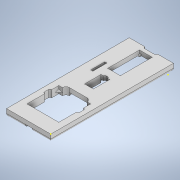
# Autodesk Inventor part: inside
Saved by Autodesk Inventor 2022 (Build 260153000, 153)
## iProperties
Created: 2022-12-24
Part Number: inside
Material: Generic
Document SubType Name: Modeling
Designer: matys
Density: 1 g/cm^3
Appearance: Default
Author: matys
Autodesk Inventor part; units mm, degrees
ref_plane "YZ Plane" through (0, 0, 0) normal (1, 0, 0) x (0, 1, 0)
ref_plane "XZ Plane" through (0, 0, 0) normal (0, 1, 0) x (-1, 0, 0)
sketch "Sketch1" plane through (0, 0, 0) normal (0, 1, 0) x (-1, 0, 0)
  line L0 (0, 0) -> (0, -173.4)
  line L1 (0, -173.4) -> (62.5, -173.4)
  line L2 (62.5, -173.4) -> (62.5, 0)
  line L3 (62.5, 0) -> (0, 0)
  dimension "d0" = 173.4
  dimension "d1" = 62.5
  constraints: 8 end point, 3 perpendicular, 1 vertical
  measures "d0" distance of L0.start L0.end
  measures "d1" distance of L0.end L1.end
extrude "Extrusion1" add sketch "Sketch1" along normal blind 10
sketch "Sketch2" plane through (0, 10, 0) normal (0, 1, 0) x (1, 0, 0)
  line L0 (0, 0) -> (0, 102.12)
  line L1 (0, 0) -> (0, 173.4) projected
  line L2 (0, 102.12) -> (-62.5, 102.12)
  line L3 (-62.5, 173.4) -> (-62.5, 0) projected
  line L4 (-31.25, 102.12) -> (-31.25, 0)
  line L5 (-62.5, 0) -> (0, 0) projected
  line L6 (-31.25, 102.12) -> (-37.45, 102.12)
  line L7 (-37.45, 102.12) -> (-31.25, 102.12)
  line L8 (-31.25, 102.12) -> (-25.05, 102.12)
  line L9 (-25.05, 102.12) -> (-31.25, 102.12)
  line L10 (-31.25, 102.12) -> (-31.25, 85.22)
  line L11 (-31.25, 85.22) -> (-25.05, 85.22)
  line L12 (-25.05, 85.22) -> (-25.05, 102.12)
  line L13 (-31.25, 85.22) -> (-37.45, 85.22)
  line L14 (-37.45, 85.22) -> (-37.45, 102.12)
  line L15 (-31.25, 102.12) -> (-31.25, 108.42)
  line L16 (-31.25, 108.42) -> (-25.05, 108.42)
  line L17 (-25.05, 108.42) -> (-25.05, 102.12)
  line L18 (-37.45, 102.12) -> (-37.45, 108.42)
  line L19 (-37.45, 108.42) -> (-31.25, 108.42)
  line L20 (-31.25, 108.42) -> (-31.25, 173.4)
  line L21 (0, 173.4) -> (-62.5, 173.4) projected
  line L22 (-31.25, 140.91) -> (-31.25, 120.66)
  line L23 (-31.25, 120.66) -> (-22.25, 120.66)
  line L24 (-22.25, 120.66) -> (-22.25, 165.66)
  line L25 (-22.25, 165.66) -> (-40.25, 165.66)
  line L26 (-40.25, 165.66) -> (-40.25, 120.66)
  line L27 (-40.25, 120.66) -> (-31.25, 120.66)
  line L28 (-40.25, 120.66) -> (-40.25, 126.66)
  line L29 (-40.25, 126.66) -> (-44.25, 126.66)
  line L30 (-44.25, 126.66) -> (-47.25, 126.66)
  line L31 (-47.25, 126.66) -> (-47.25, 106.66)
  line L32 (-47.25, 106.66) -> (-50.25, 106.66)
  line L33 (-50.25, 106.66) -> (-50.25, 126.66)
  line L34 (-50.25, 126.66) -> (-47.25, 126.66)
  line L35 (-31.25, 0) -> (-31.25, 85.22)
  line L36 (-31.25, 42.61) -> (-31.25, 20.11)
  line L37 (-31.25, 20.11) -> (-31.25, 42.61)
  line L38 (-31.25, 42.61) -> (-31.25, 65.11)
  line L39 (-31.25, 65.11) -> (-53.75, 65.11)
  line L40 (-53.75, 65.11) -> (-53.75, 20.11)
  line L41 (-53.75, 20.11) -> (-8.75, 20.11)
  line L42 (-8.75, 20.11) -> (-8.75, 65.11)
  line L43 (-8.75, 65.11) -> (-31.25, 65.11)
  line L44 (-22.25, 120.66) -> (-40.25, 120.66)
  line L45 (-40.25, 120.66) -> (-40.25, 165.66)
  line L46 (-40.25, 165.66) -> (-22.25, 165.66)
  line L47 (-22.25, 165.66) -> (-22.25, 120.66)
  line L48 (-53.75, 65.11) -> (-48.75, 65.11)
  line L49 (-48.75, 65.11) -> (-8.75, 65.11)
  line L50 (-8.75, 65.11) -> (-13.75, 65.11)
  line L51 (-13.75, 65.11) -> (-13.75, 70.11)
  line L52 (-13.75, 70.11) -> (-48.75, 70.11)
  line L53 (-48.75, 70.11) -> (-48.75, 65.11)
  line L54 (-48.75, 65.11) -> (-13.75, 65.11) construction
  line L55 (-18.75, 70.11) -> (-43.75, 70.11)
  arc A0 (-43.75, 70.11) -> (-48.75, 65.11) centre (-43.75, 65.11) ccw
  arc A1 (-13.75, 65.11) -> (-18.75, 70.11) centre (-18.75, 65.11) ccw
  line L56 (-8.75, 65.11) -> (-8.75, 55.11)
  line L57 (-8.75, 55.11) -> (-8.75, 45.11)
  line L58 (-8.75, 45.11) -> (-53.75, 45.11)
  line L59 (-53.75, 45.11) -> (-53.75, 55.11)
  line L60 (-53.75, 45.11) -> (-53.75, 55.11) construction
  line L61 (-51.25, 47.61) -> (-51.25, 52.61)
  line L62 (-56.25, 52.61) -> (-56.25, 47.61)
  arc A2 (-56.25, 47.61) -> (-51.25, 47.61) centre (-53.75, 47.61) ccw
  arc A3 (-51.25, 52.61) -> (-56.25, 52.61) centre (-53.75, 52.61) ccw
  line L63 (-8.75, 45.11) -> (-8.75, 55.11) construction
  line L64 (-6.25, 47.61) -> (-6.25, 52.61)
  line L65 (-11.25, 52.61) -> (-11.25, 47.61)
  arc A4 (-11.25, 47.61) -> (-6.25, 47.61) centre (-8.75, 47.61) ccw
  arc A5 (-6.25, 52.61) -> (-11.25, 52.61) centre (-8.75, 52.61) ccw
  line L66 (-40.25, 165.66) -> (-40.25, 173.4)
  line L67 (-22.25, 165.66) -> (-22.25, 173.4)
  line L68 (-40.25, 173.4) -> (-22.25, 173.4) construction
  line L69 (-37.75, 170.9) -> (-24.75, 170.9)
  line L70 (-24.75, 175.9) -> (-37.75, 175.9)
  arc A6 (-37.75, 175.9) -> (-37.75, 170.9) centre (-37.75, 173.4) ccw
  arc A7 (-24.75, 170.9) -> (-24.75, 175.9) centre (-24.75, 173.4) ccw
  line L71 (-31.25, 102.12) -> (-34.35, 102.12)
  line L72 (-28.15, 102.12) -> (-31.25, 102.12)
  line L73 (-34.35, 102.12) -> (-28.15, 102.12) construction
  line L74 (-32.35, 100.12) -> (-30.15, 100.12)
  line L75 (-30.15, 104.12) -> (-32.35, 104.12)
  arc A8 (-32.35, 104.12) -> (-32.35, 100.12) centre (-32.35, 102.12) ccw
  arc A9 (-30.15, 100.12) -> (-30.15, 104.12) centre (-30.15, 102.12) ccw
  arc A10 (-32.35, 110.42) -> (-32.35, 106.42) centre (-32.35, 108.42) ccw
  arc A11 (-30.15, 106.42) -> (-30.15, 110.42) centre (-30.15, 108.42) ccw
  line L76 (-32.35, 110.42) -> (-30.15, 110.42)
  point P0 (-31.25, 165.66)
  point P1 (-31.25, 165.66)
  point P2 (-53.75, 50.11)
  point P3 (-8.75, 50.11)
  point P4 (-34.35, 108.42)
  point P5 (-28.15, 108.42)
  dimension "d4" = 102.12
  dimension "d5" = 6.2
  dimension "d6" = 6.2
  dimension "d7" = 16.9
  dimension "d8" = 6.3
  dimension "d11" = 20.25
  dimension "d12" = 9
  dimension "d13" = 45
  dimension "d14" = 18
  dimension "d15" = 6
  dimension "d16" = 4
  dimension "d17" = 3
  dimension "d18" = 20
  dimension "d19" = 3
  dimension "d20" = 22.5
  dimension "d21" = 22.5
  dimension "d22" = 22.5
  dimension "d23" = 45
  dimension "d24" = 5
  dimension "d25" = 5
  dimension "d26" = 5
  dimension "d27" = 10
  dimension "d28" = 10
  dimension "d29" = 5
  dimension "d30" = 5
  dimension "d36" = 5
  dimension "d37" = 4
  dimension "d39" = 4
  constraints: 156 end point, 35 point on circle, 33 point on line, 30 perpendicular, 18 tangent, 12 centre point, 12 midpoint, 7 collinear, 7 parallel, 4 horizontal, 1 vertical
  measures "d4" distance of L0.start L0.end
  measures "d5" distance of L4.start L6.end
  measures "d6" distance of L4.start L8.end
  measures "d7" distance of L4.start L10.end
  measures "d8" distance of L4.start L15.end
  measures "d11" distance of L22.start L22.end
  measures "d12" distance of L22.end L23.end
  measures "d13" distance of L23.end L24.end
  measures "d14" distance of L24.end L25.end
  measures "d15" distance of L26.end L28.end
  measures "d16" distance of L28.end L29.end
  measures "d17" distance of L29.end L30.end
  measures "d18" distance of L30.end L31.end
  measures "d19" distance of L31.end L32.end
  measures "d20" distance of L36.start L36.end
  measures "d21" distance of L36.start L38.end
  measures "d22" distance of L38.end L39.end
  measures "d23" distance of L40.end L41.end
  measures "d24" distance of L48.end L39.end
  measures "d25" distance of L50.end L42.end
  measures "d26" distance of L50.end L51.end
  measures "d27" distance of L42.end L56.end
  measures "d28" distance of L56.end L57.end
  measures "d29" diameter of A3
  measures "d30" diameter of A5
  measures "d36" diameter of A7
  measures "d37" diameter of A9
  measures "d39" diameter of A11
extrude "Extrusion2" cut sketch "Sketch2" against normal through all contours L12 L11 L4 L74 A9 L2 | L2 A9 L75 L15 L16 L17 | L41 L40 L58 L4 | L4 L58 L42 L41 | A7 L69 L20 L21 | A9 L74 L4 L2 | L2 L15 L75 A9 | L31 L32 L33 L34 | L20 L69 A6 L21 | L24 L23 L20 L25 | L4 L74 A8 L2 | L2 A8 L75 L15 | L13 L14 L2 A8 L74 L4 | L16 L20 L76 A11 | L58 A2 L61 A3 L40 L39 L4 | L4 L43 L42 A5 L65 A4 L58 | A2 L62 A3 L40 | L40 A3 L61 A2 | A4 L65 A5 L42 | L42 A5 L64 A4 | L18 L19 L15 L75 A8 L2 | L20 L27 L26 L25 | L52 A1 L43 L4 | L4 L39 A0 L52 | L19 A10 L76 L20
sketch "Sketch3" plane through (0, 10, 0) normal (0, 1, 0) x (1, 0, 0)
  point P0 (0, 0)
sketch "Sketch4" plane through (0, 0, 0) normal (0, -1, 0) x (1, 0, 0)
  line L0 (-8.75, -20.11) -> (-53.75, -20.11) projected
  line L1 (-53.75, -20.11) -> (-8.75, -20.11)
  line L2 (-8.75, -20.11) -> (-31.25, -20.11)
  line L3 (-62.5, 0) -> (0, 0) projected
  line L4 (-31.25, 0) -> (-31.25, -20.11)
  line L5 (-31.25, -20.11) -> (-26.25, -20.11)
  line L6 (-26.25, -20.11) -> (-36.25, -20.11)
  line L7 (-36.25, -20.11) -> (-36.25, 0)
  line L8 (-36.25, 0) -> (-26.25, 0)
  line L9 (-26.25, 0) -> (-26.25, -20.11)
  line L10 (-40.25, -165.66) -> (-40.25, -120.66) projected
  line L11 (-40.25, -120.66) -> (-47.25, -120.66)
  line L12 (-47.25, -126.66) -> (-47.25, -106.66) projected
  line L13 (-48.8082, -126.9328) -> (-40.25, -126.9328)
  line L14 (-40.25, -126.9328) -> (-48.8082, -126.9328)
  line L15 (-40.25, -165.66) -> (-22.25, -165.66) projected
  line L16 (-40.25, -165.66) -> (-48.8082, -165.66)
  line L17 (-48.8082, -165.66) -> (-48.8082, -126.9328)
  line L18 (-22.25, -120.66) -> (-22.25, -165.66) projected
  line L19 (-22.25, -165.66) -> (-15.25, -165.66)
  line L20 (-15.25, -165.66) -> (-15.25, -120.66)
  line L21 (-15.25, -120.66) -> (-22.25, -120.66)
  line L22 (-40.25, -120.66) -> (-22.25, -120.66) projected
  line L23 (-22.25, -120.66) -> (-40.25, -120.66)
  line L24 (-40.25, -120.66) -> (-40.25, -126.9328)
  line L25 (-40.25, -165.66) -> (-40.25, -126.9328)
  line L26 (-22.25, -120.66) -> (-22.25, -165.66)
  line L27 (-40.25, -165.66) -> (-40.25, -173.4)
  line L28 (0, -173.4) -> (-62.5, -173.4) projected
  line L29 (-48.8082, -165.66) -> (-40.25, -173.4)
  line L30 (-22.25, -165.66) -> (-22.25, -173.4)
  line L31 (-22.25, -173.4) -> (-15.25, -165.66)
  line L32 (-40.25, -173.4) -> (-22.25, -173.4)
  line L33 (-37.45, -108.42) -> (-37.45, -85.22) projected
  line L34 (-25.05, -85.22) -> (-25.05, -108.42) projected
  line L35 (-37.45, -108.42) -> (-25.05, -108.42)
  line L36 (-25.05, -108.42) -> (-22.25, -120.66)
  line L37 (-37.45, -108.42) -> (-40.25, -120.66)
  line L38 (-43.75, -70.11) -> (-18.75, -70.11) projected
  line L39 (-50.25, -126.66) -> (-50.25, -106.66) projected
  line L40 (-43.75, -70.11) -> (-50.25, -106.66)
  line L41 (-47.25, -106.66) -> (-50.25, -106.66) projected
  line L42 (-47.25, -106.66) -> (-40.25, -70.11)
  line L43 (-18.75, -70.11) -> (-15.25, -120.66)
  line L44 (-25.05, -108.42) -> (-37.45, -108.42) projected
  line L45 (-25.05, -85.22) -> (-37.45, -85.22) projected
  line L46 (-25.05, -108.42) -> (-25.05, -85.22)
  line L47 (-25.05, -85.22) -> (-43.1438, -85.22)
  line L48 (-37.45, -108.42) -> (-47.25, -120.66)
  line L49 (-48.8082, -126.9328) -> (-48.8082, -120.66)
  line L50 (-48.8082, -120.66) -> (-47.25, -120.66)
  line L51 (-37.45, -108.42) -> (-47.25, -108.42)
  line L52 (-37.45, -108.42) -> (-38.0612, -111.0919)
  line L53 (-38.0612, -111.0919) -> (-47.25, -111.0919)
  point P0 (-39.5893, -111.0919)
  dimension "d31" = 5
  dimension "d32" = 10
  dimension "d33" = 7
  constraints: 78 end point, 14 perpendicular, 13 point on line, 4 horizontal, 3 collinear, 2 midpoint, 2 vertical, 1 parallel
  measures "d31" distance of L2.end L5.end
  measures "d32" distance of L5.end L6.end
  measures "d33" distance of L15.end L19.end
extrude "Extrusion3" cut sketch "Sketch4" against normal blind 4 contours L0 L4 L3 L9 | L0 L7 L3 L4 | L16 L17 L13 L10 | L27 L29 L16 | L15 L30 L28 L27 | L13 L49 L50 L11 L10 | L18 L21 L20 L19 | L19 L31 L30 | L37 L35 L36 L22 | L11 L48 L53 L37 | L36 L34 L45 L47 L42 L38 L43 L21 | L53 L48 L37 | L12 L51 L48 L53 | L42 L41 L40 L38
sketch "Sketch5" plane through (-40.25, 10, -165.66) normal (0, 0, 1) x (1, 0, 0)
  point P0 (40.25, -10)
fillet "Fillet1" radius 4 6 edges at (0, 0, -86.7) (-62.5, 0, -86.7) (-49.375, 0, 0) (-13.125, 0, 0) (-51.375, 0, -173.4) (-11.125, 0, -173.4)
ref_plane "Work Plane1" through (-38.25, 4, -70.11) normal (0, -1, 0) x (1, 0, 0)
sketch "Sketch6" plane through (-38.25, 4, -70.11) normal (0, -1, 0) x (1, 0, 0)
  line L0 (-15.5, 15) -> (-15.5, 5) projected
  arc A0 (-10.5, 5) -> (-5.5, 0) centre (-5.5, 5) ccw projected
  line L1 (-15.5, 5) -> (-10.5, 5)
  line L2 (-15.5, 5) -> (-10.5, 5) projected
  line L3 (-10.5, 5) -> (-15.5, 5)
  line L4 (-15.5, 5) -> (-15.5, 10)
  line L5 (-15.5, 10) -> (-10.5, 5)
  line L6 (-15.5, 50) -> (-15.5, 25) projected
  line L7 (-15.5, 50) -> (-15.5, 45)
  line L8 (-15.5, 45) -> (-15.5, 50)
  line L9 (-15.5, 50) -> (2, 50) projected
  line L10 (-15.5, 50) -> (-10.5, 50)
  line L11 (-10.5, 50) -> (-15.5, 45)
  line L12 (-5.5, 0) -> (19.5, 0) projected
  line L13 (7, 0) -> (7, 50)
  line L14 (12, 50) -> (2, 50) projected
  line L15 (29.5, 15) -> (29.5, 5)
  line L16 (29.5, 5) -> (24.5, 5)
  line L17 (29.5, 10) -> (24.5, 5)
  line L18 (29.5, 50) -> (29.5, 45)
  line L19 (29.5, 50) -> (12, 50)
  line L20 (24.5, 50) -> (29.5, 45)
  line L21 (-2, -50.55) -> (-2, -95.55) projected
  line L22 (-2, -50.55) -> (-2, -53.05)
  line L23 (-2, -53.05) -> (-2, -50.55)
  line L24 (-2, -50.55) -> (-2, -53.05)
  line L25 (-2, -53.05) -> (0.5, -53.05)
  line L26 (0.5, -53.05) -> (0.5, -50.55)
  line L27 (16, -50.55) -> (-2, -50.55) projected
  line L28 (-2, -50.55) -> (0.5, -50.55)
  line L29 (-2, -50.55) -> (-2, -53.05)
  line L30 (7, -50.55) -> (7, -95.55)
  line L31 (-2, -95.55) -> (16, -95.55) projected
  line L32 (-2, -95.55) -> (-2, -93.05)
  line L33 (-2, -93.05) -> (0.5, -93.05)
  line L34 (0.5, -93.05) -> (0.5, -95.55)
  line L35 (0.5, -95.55) -> (-2, -95.55)
  line L36 (16, -50.55) -> (16, -95.55)
  line L37 (16, -50.55) -> (16, -53.05)
  line L38 (16, -53.05) -> (13.5, -53.05)
  line L39 (13.5, -53.05) -> (13.5, -50.55)
  line L40 (-2, -50.55) -> (16, -50.55)
  line L41 (16, -95.55) -> (-2, -95.55)
  line L42 (16, -93.05) -> (13.5, -93.05)
  line L43 (13.5, -93.05) -> (13.5, -95.55)
  point P0 (38.25, 70.11)
  dimension "d40" = 5
  dimension "d41" = 5
  dimension "d42" = 5
  dimension "d43" = 2.5
  dimension "d44" = 2.5
  dimension "d45" = 2.5
  dimension "d46" = 2.5
  constraints: 70 end point, 17 symmetric about line, 15 point on line, 4 collinear, 4 perpendicular, 3 midpoint, 2 horizontal
  measures "d40" distance of L0.end L4.end
  measures "d41" distance of L6.start L7.end
  measures "d42" distance of L6.start L10.end
  measures "d43" distance of L21.start L22.end
  measures "d44" distance of L22.end L23.end
  measures "d45" distance of L22.end L25.end
  measures "d46" distance of L21.end L32.end
extrude "Extrusion4" add sketch "Sketch6" against normal blind 2 contours L5 L1 L0 | L11 L6 L9 | L19 L18 L20 | L15 L16 L17 | L27 L26 L25 L21 | L33 L34 L31 L21 | L27 L36 L38 L39 | L43 L42 L36 L31
chamfer "Chamfer1" distance 3.535 distance2 2 1 edges at (-51.25, 6, -22.61) measured on face at (-52.0833, 6, -21.7767)
chamfer "Chamfer2" distance 3.535 distance2 2 1 edges at (-51.25, 6, -62.61) measured on face at (-52.0833, 6, -63.4433)
chamfer "Chamfer3" distance 3.535 distance2 2 1 edges at (-11.25, 6, -62.61) measured on face at (-10.4167, 6, -63.4433)
chamfer "Chamfer4" distance 3.535 distance2 2 1 edges at (-11.25, 6, -22.61) measured on face at (-10.4167, 6, -21.7767)
chamfer "Chamfer5" distance 2.5 distance2 2 1 edges at (-23.5, 6, -123.16) measured on face at (-23.0833, 6, -122.3267)
chamfer "Chamfer6" distance 2.5 distance2 2 1 edges at (-39, 6, -123.16) measured on face at (-39.4167, 6, -121.4933)
chamfer "Chamfer7" distance 2.5 distance2 2 1 edges at (-39, 6, -163.16) measured on face at (-39.4167, 6, -163.9933)
chamfer "Chamfer8" distance 2.5 distance2 2 1 edges at (-23.5, 6, -163.16) measured on face at (-23.9167, 6, -163.9933)
body "Solid1"
